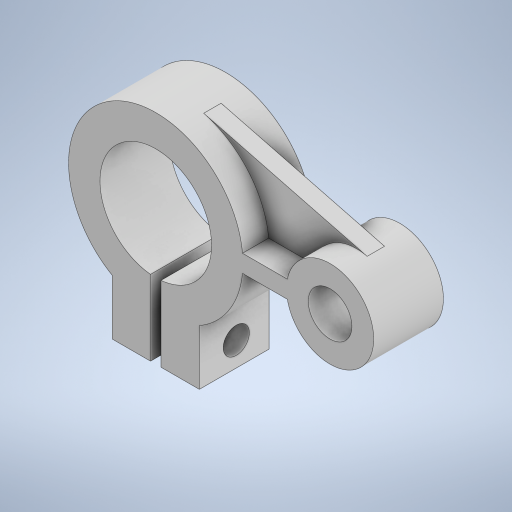
# Autodesk Inventor part: 5
Saved by Autodesk Inventor 2023 (Build 270158000, 158)
## iProperties
Created: 2023-10-17
Part Number: 5
Material: Všeobecné
Document SubType Name: Modeling
Designer: clu40164
Mass: 303.589 g
Surface Area: 552.649 cm^2
Volume: 303.589 cm^3
Density: 1 g/cm^3
Appearance: Výchozí
Author: clu40164
Autodesk Inventor part; units mm, degrees
ref_plane "YZ Plane" through (0, 0, 0) normal (1, 0, 0) x (0, 1, 0)
ref_plane "XZ Plane" through (0, 0, 0) normal (0, 1, 0) x (-1, 0, 0)
ref_plane "XY Plane" through (0, 0, 0) normal (0, 0, 1) x (1, 0, 0)
sketch "Náčrt1" plane through (0, 0, 0) normal (0, 0, 1) x (1, 0, 0)
  arc A0 (3, -31.8591) -> (-3, -31.8591) centre (0, 0) ccw
  circle A1 centre (100, 0) radius 12.5
  arc A2 (75.5051, -5) -> (75.5051, 5) centre (100, 0) ccw
  line L0 (12.5, 48.4123) -> (106.25, 24.2061)
  line L1 (49.7494, 5) -> (75.5051, 5)
  line L2 (75.5051, -5) -> (49.7494, -5)
  line L3 (3, -75) -> (25, -75)
  line L4 (-3, -75) -> (-25, -75)
  line L5 (-25, -75) -> (-25, -43.3013)
  line L6 (25, -75) -> (25, -43.3013)
  line L7 (3, -75) -> (3, -31.8591)
  line L8 (-3, -75) -> (-3, -31.8591)
  arc A3 (25, -43.3013) -> (49.7494, -5) centre (0, 0) ccw
  arc A4 (49.7494, 5) -> (-25, -43.3013) centre (0, 0) ccw
  dimension "d1" = 64
  dimension "d3" = 25
  dimension "d4" = 50
  dimension "d9" = 10
  dimension "d10" = 22
  dimension "d11" = 22
  dimension "d12" = 6
  constraints: 18 end point, 10 point on circle, 5 centre point, 3 coincident, 2 tangent, 1 horizontal, 1 parallel, 1 perpendicular
  measures "d1" diameter of A0
  measures "d3" diameter of A1
  measures "d4" diameter of A2
  measures "d9" distance between parallel lines of L2 L1
  measures "d10" distance of L4.start L4.end
  measures "d11" distance of L3.start L3.end
  measures "d12" distance of L3.start L4.start
extrude "Vysunutí1" add sketch "Náčrt1" against normal blind 20 contours A0 L8 L4 L5 A4 L1 A2 L2 A3 L6 L3 L7
extrude "Vysunutí2" add sketch "Náčrt1" against normal blind 5 contours L0 A2 L1 A4
extrude "Vysunutí3" add sketch "Náčrt1" along normal blind 5 contours L0 A2 L1 A4
extrude "Vysunutí4" add sketch "Náčrt1" along normal blind 20 contours A0 L8 L4 L5 A4 L1 A2 L2 A3 L6 L3 L7
sketch "Náčrt2" plane through (25, -75, -20) normal (1, 0, 0) x (0, 0, -1)
  point P0 (-20, 75)
  point P1 (-18.8172, 13.7965)
hole "Díra1" at (25, -61.2035, -1.1828) direction (-1, 0, 0) diameter 15 end through all
